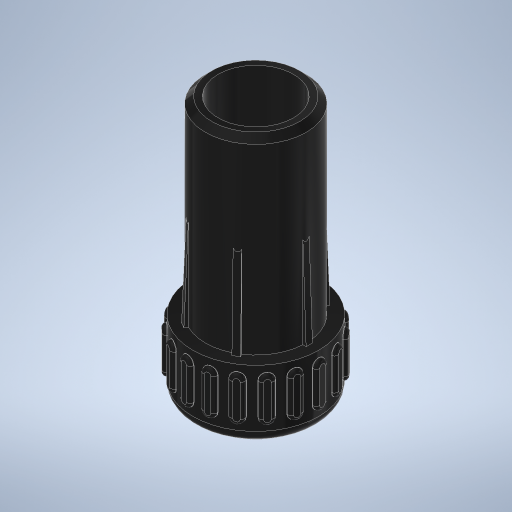
# Autodesk Inventor part: Plastic tube in support
Saved by Autodesk Inventor 2024 (Build 280153000, 153)
## iProperties
Created: 2013-11-20
Part Number: Plastic tube in support
Material: Plastic, Opaque Black
Document SubType Name: Modeling
Designer: SauliusD
Density: 0.952 g/cm^3
Appearance: Smooth - Black
Author: SauliusD
Autodesk Inventor part; units mm, degrees
ref_plane "YZ Plane" through (0, 0, 0) normal (1, 0, 0) x (0, 1, 0)
ref_plane "XZ Plane" through (0, 0, 0) normal (0, 1, 0) x (-1, 0, 0)
ref_plane "XY Plane" through (0, 0, 0) normal (0, 0, 1) x (1, 0, 0)
sketch "Sketch1" plane through (0, 0, 0) normal (0, 0, 1) x (1, 0, 0)
  circle A0 centre (0, 0) radius 8
  dimension "d0" = 16
  constraints: 1 centre point, 1 coincident
  measures "d0" diameter of A0
extrude "Extrusion1" add sketch "Sketch1" along normal blind 30
shell "Shell1" thickness 2 removed faces 1 at (3.8323, 2.2209, 30)
sketch "Sketch2" plane through (0, 0, 0) normal (0, 0, -1) x (-1, 0, 0)
  circle A0 centre (0, 0) radius 8 projected
  circle A1 centre (0, 0) radius 10
  dimension "d3" = 2
  constraints: 1 centre point
  measures "d3" radial gap between concentric circles of A1 A0
extrude "Extrusion2" add sketch "Sketch2" along normal blind 10 contours A0 | A1
sketch "Sketch3" plane through (0, 0, 0) normal (0, 1, 0) x (-1, 0, 0)
  line L0 (-10, -10) -> (10, -10) projected
  arc A0 (-10, -10) -> (0, -14) centre (0, 0.5) ccw
  line L1 (0, -14) -> (0, -10)
  line L2 (-10, -10) -> (0, -10)
  point P0 (0, 0)
  dimension "d6" = 4
  constraints: 4 end point, 2 point on circle, 2 vertical alignment, 1 centre point, 1 collinear, 1 midpoint
  measures "d6" distance of L1.start L1.end
revolve "Revolution1" add sketch "Sketch3" angle 360 about axis through (0, 0, -14) along (0, 0, 1)
chamfer "Chamfer1" distance 1 angle 45 1 edges at (-8, 0, 30)
fillet "Fillet1" radius 2 2 edges at (0, -10, -10) (0, 10, -10)
sketch "Sketch4" plane through (0, 0, 0) normal (0, 1, 0) x (-1, 0, 0)
  line L0 (-10, 0) -> (-10, -9.1047) construction
  line L1 (-9.4, -1) -> (-10.6, -1)
  line L2 (-10.6, -1) -> (-10.6, -8.1047)
  line L3 (-10.6, -8.1047) -> (-9.4, -8.1047)
  line L4 (-9.4, -8.1047) -> (-9.4, -1)
  line L5 (10, 0) -> (-10, 0) projected
  point P0 (0, 0)
  dimension "d13" = 0.6
  dimension "d14" = 1
  dimension "d15" = 1
  constraints: 8 end point, 2 parallel, 1 horizontal, 1 perpendicular, 1 other
  measures "d14" distance between parallel lines of L5 L1
  measures "d15" distance from line of L0.end L3
extrude "Extrusion3" add sketch "Sketch4" along normal mid plane 2
fillet "Fillet2" radius 1 4 edges at (10.2749, 1, -1) (10.2749, 1, -8.1047) (10.2749, -1, -8.1047) (10.2749, -1, -1)
fillet "Fillet3" radius 0.56 4 edges at (10.6, 0.7073, -1.2927) (10.6, 1, -4.5523) (10.6, 0.7073, -7.8119) (10.6, -1, -4.5523)
pattern_circular "Circular Pattern1" count 19 over 360 about axis through (0, 0, -10) along (0, 0, 1) of "Extrusion3", "Fillet2", "Fillet3"
sketch "Sketch5" plane through (0, 0, 0) normal (0, 1, 0) x (-1, 0, 0)
  line L0 (-8, 0) -> (-8, 29) construction
  line L1 (-7.5, 28) -> (-8.5, 0)
  line L2 (-8.5, 0) -> (-7.5, 0)
  line L3 (-7.5, 0) -> (-7.5, 28)
  point P0 (0, 0)
  point P1 (-8, 14)
  dimension "d23" = 14
  dimension "d24" = 0.5
  constraints: 6 end point, 2 midpoint, 1 perpendicular, 1 vertical
  measures "d23" distance from line of L2 point (-8, 14)
  measures "d24" distance from line of L0 L1.end
extrude "Extrusion4" add sketch "Sketch5" along normal mid plane 1
pattern_circular "Circular Pattern2" count 6 over 360 about axis through (0, 0, -10) along (0, 0, 1) of "Extrusion4"
body "Solid1"
